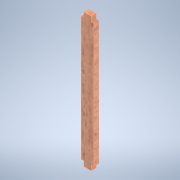
# Autodesk Inventor part: MagnetHolder
Saved by Autodesk Inventor 2022.2 (Build 262287000, 287)
## iProperties
Created: 2023-02-28
Part Number: MagnetHolder
Material: Wood (Oak)
Document SubType Name: Modeling
Designer: jaege
Density: 0.76 g/cm^3
Appearance: Red Oak - Natural Low Gloss
Author: jaege
Autodesk Inventor part; units mm, degrees
ref_plane "YZ Plane" through (0, 0, 0) normal (1, 0, 0) x (0, 1, 0)
ref_plane "XZ Plane" through (0, 0, 0) normal (0, 1, 0) x (-1, 0, 0)
ref_plane "XY Plane" through (0, 0, 0) normal (0, 0, 1) x (1, 0, 0)
sketch "Sketch1" plane through (0, 0, 0) normal (0, 0, 1) x (1, 0, 0)
  line L0 (3, 54) -> (-3, 54)
  line L1 (-3, 54) -> (-3, 50)
  line L2 (-3, -54) -> (3, -54)
  line L3 (3, -54) -> (3, -50)
  line L4 (-3, 50) -> (-5, 50)
  line L5 (-5, 50) -> (-5, -50)
  line L6 (-5, -50) -> (-3, -50)
  line L7 (-3, -50) -> (-3, 50) construction
  line L8 (-3, 50) -> (-3, -50) construction
  line L9 (-3, -50) -> (-3, -54)
  line L10 (0, 54) -> (0, -54)
  line L11 (3, 50) -> (5, 50)
  line L12 (5, 50) -> (5, -50)
  line L13 (5, -50) -> (3, -50)
  line L14 (3, 50) -> (3, 54)
  line L15 (3, -50) -> (3, 50) construction
  point P0 (0, 0)
  point P1 (-4, -50)
  point P2 (0, 0)
  point P3 (0, 0)
  dimension "d0" = 6
  dimension "d1" = 108
  dimension "d2" = 4
  dimension "d3" = 4
  dimension "d4" = 2
  constraints: 32 end point, 15 parallel, 4 midpoint, 4 perpendicular, 4 symmetric about line, 2 coincident, 2 horizontal
  measures "d0" distance of L0.start L0.end
  measures "d1" distance of L2.end L0.start
  measures "d2" distance from line of L10.start L4
  measures "d3" horizontal distance of L10.end point (-4, -50)
  measures "d4" distance of L1.end L4.end
extrude "Extrusion1" add sketch "Sketch1" along normal blind 4
body "Solid1"
